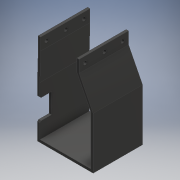
# Autodesk Inventor part: nema 17 holder
Saved by Autodesk Inventor 2018 (Build 220112000, 112)
## iProperties
Created: 2017-11-24
Part Number: nema 17 holder
Material: Acetal Resin, Black
Document SubType Name: Modeling
Designer: g
Density: 1.425 g/cm^3
Appearance: Smooth - Black
Author: g
Autodesk Inventor part; units mm, degrees
ref_plane "YZ Plane" through (0, 0, 0) normal (1, 0, 0) x (0, 1, 0)
ref_plane "XZ Plane" through (0, 0, 0) normal (0, 1, 0) x (-1, 0, 0)
ref_plane "XY Plane" through (0, 0, 0) normal (0, 0, 1) x (1, 0, 0)
sketch "Sketch3" plane through (0, 0, 0) normal (0, 1, 0) x (-1, 0, 0)
  line L0 (0, 0) -> (15, 0) construction
  line L1 (0, 0) -> (-15, 0) construction
  line L2 (15, 0) -> (15, -10)
  line L3 (15, -10) -> (17, -10)
  line L4 (17, -10) -> (17, 0)
  line L5 (17, 0) -> (15, 0)
  line L6 (-15, 0) -> (-15, -10)
  line L7 (-15, -10) -> (-17, -10)
  line L8 (-17, -10) -> (-17, 0)
  line L9 (-17, 0) -> (-15, 0)
  line L10 (0, 0) -> (0, -74) construction
  line L11 (0, -74) -> (15.65, -74)
  line L12 (0, -74) -> (-26.65, -74)
  line L13 (15.65, -74) -> (15.65, -76)
  line L14 (15.65, -76) -> (-26.65, -76)
  line L15 (-26.65, -76) -> (-26.65, -74)
  line L16 (15.65, -76) -> (17.65, -76)
  line L17 (17.65, -76) -> (17.65, -33)
  line L18 (17.65, -33) -> (17, -10)
  line L19 (-26.65, -76) -> (-28.65, -76)
  line L20 (-28.65, -76) -> (-28.65, -33)
  line L21 (-28.65, -33) -> (-17, -10)
  line L22 (-26.65, -33) -> (-26.65, -74)
  line L23 (-26.65, -33) -> (-15, -10)
  line L24 (15.65, -74) -> (15.65, -33)
  line L25 (15.65, -33) -> (15, -10)
  dimension "d19" = 15
  dimension "d20" = 15
  dimension "d21" = 10
  dimension "d22" = 2
  dimension "d23" = 2
  dimension "d24" = 74
  dimension "d25" = 15.65
  dimension "d26" = 26.65
  dimension "d27" = 2
  dimension "d28" = 2
  dimension "d29" = 43
  dimension "d30" = 2
  constraints: 52 end point, 11 perpendicular, 5 point on line, 4 horizontal, 4 vertical
  measures "d19" distance of L0.start L0.end
  measures "d20" distance of L0.start L1.end
  measures "d21" distance of L0.end L2.end
  measures "d22" distance of L2.end L3.end
  measures "d23" distance of L6.end L7.end
  measures "d24" distance of L0.start L10.end
  measures "d25" distance of L10.end L11.end
  measures "d26" distance of L10.end L12.end
  measures "d27" distance of L11.end L13.end
  measures "d28" distance of L13.end L16.end
  measures "d29" distance of L16.end L17.end
  measures "d30" distance of L14.end L19.end
extrude "Extrusion3" add sketch "Sketch3" along normal blind 41
sketch "Sketch4" plane through (17, 0, 0) normal (1, 0, 0) x (0, 0, -1)
  line L0 (0, 41) -> (10, 41) projected
  line L1 (5, 41) -> (5, 0) construction
  line L2 (0, 0) -> (10, 0) projected
  circle A0 centre (5, 36) radius 1.5
  circle A1 centre (5, 21) radius 1.5
  circle A2 centre (5, 5) radius 1.5
  dimension "d33" = 3
  dimension "d34" = 3
  dimension "d35" = 3
  dimension "d36" = 5
  dimension "d37" = 20
  dimension "d38" = 5
  constraints: 3 centre point, 3 point on line, 2 end point, 2 midpoint
  measures "d33" diameter of A0
  measures "d34" diameter of A1
  measures "d35" diameter of A2
  measures "d36" distance from line of L2 A2.centre
  measures "d37" distance from line of L0 A1.centre
  measures "d38" distance from line of L0 A0.centre
extrude "Extrusion4" cut sketch "Sketch4" against normal blind 41
sketch "Sketch5" plane through (-15.65, 0, -33) normal (1, 0, 0) x (0, 0, -1)
  line L0 (43, 41) -> (0, 41) construction
  line L1 (43, 41) -> (28, 41) construction
  line L2 (28, 41) -> (11.3, 41)
  line L3 (0, 41) -> (41, 41) projected
  line L4 (11.3, 41) -> (11.3, 31.2)
  line L5 (11.3, 31.2) -> (28, 31.2)
  line L6 (28, 31.2) -> (28, 41)
  line L7 (-33, 0) -> (-33, 41) projected
  line L8 (-33, 20.5) -> (43.2926, 20.5)
  line L9 (43, 0) -> (0, 0) construction
  line L10 (28, 0) -> (11.3, 0)
  line L11 (11.3, 0) -> (11.3, 9.8)
  line L12 (11.3, 9.8) -> (28, 9.8)
  line L13 (28, 9.8) -> (28, 0)
  dimension "d41" = 15
  dimension "d42" = 16.7
  dimension "d43" = 9.8
  constraints: 22 end point, 6 symmetric about line, 3 point on line, 2 perpendicular, 1 horizontal, 1 midpoint, 1 vertical
  measures "d41" distance of L0.start L1.end
  measures "d42" distance of L1.end L2.end
  measures "d43" distance of L2.end L4.end
extrude "Extrusion5" cut sketch "Sketch5" against normal blind 41 contours L10 L11 L12 L13
chamfer "Chamfer1" distance 1 angle 45 2 edges at (-16.65, 0, -61) (-16.65, 0, -44.3)
body "Solid2"
